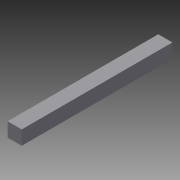
# Autodesk Inventor part: sidepeices
Saved by Autodesk Inventor 2015 (Build 190159000, 159)
## iProperties
Created: 2014-10-11
Part Number: sidepeices
Material: Generic
Document SubType Name: Modeling
Designer: jesse
Density: 1 g/cm^3
Appearance: Default
Author: jesse
Autodesk Inventor part; units mm, degrees
ref_plane "YZ Plane" through (0, 0, 0) normal (1, 0, 0) x (0, 1, 0)
ref_plane "XZ Plane" through (0, 0, 0) normal (0, 1, 0) x (-1, 0, 0)
ref_plane "XY Plane" through (0, 0, 0) normal (0, 0, 1) x (1, 0, 0)
sketch "Sketch1" plane through (0, 0, 0) normal (0, 0, 1) x (1, 0, 0)
  line L0 (0, 0) -> (19.05, 0)
  line L1 (19.05, 0) -> (19.05, 19.05)
  line L2 (19.05, 19.05) -> (0, 19.05)
  line L3 (0, 19.05) -> (0, 0)
  dimension "d0" = 19.05
  dimension "d1" = 19.05
  constraints: 8 end point, 2 parallel, 1 horizontal, 1 perpendicular
  measures "d0" distance of L2.end L1.end
  measures "d1" distance of L1.end L0.end
extrude "Extrusion1" add sketch "Sketch1" along normal blind 203.2
sketch "Sketch2" plane through (19.05, 0, 0) normal (1, 0, 0) x (0, 0, -1)
  line L0 (0, 0) -> (0, 19.05) projected
  line L1 (0, 19.05) -> (-203.2, 19.05) projected
  line L2 (-203.2, 0) -> (-203.2, 19.05) projected
  line L3 (0, 0) -> (-203.2, 0) projected
  line L4 (0, 9.525) -> (-203.2, 9.525) construction
  line L5 (-203.2, 0) -> (-203.2, 19.05) construction
  circle A0 centre (-12.6343, 9.525) radius 3.175
  dimension "d4" = 6.35
  constraints: 2 end point, 2 midpoint, 1 centre point, 1 point on line
  measures "d4" diameter of A0
extrude "Extrusion2" cut sketch "Sketch2" against normal through all contours A0
body "Solid1"
